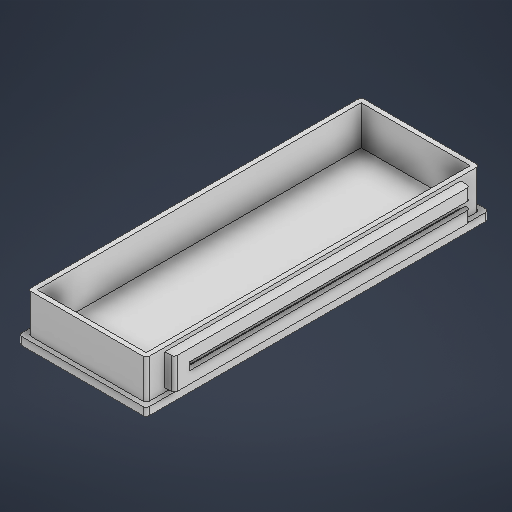
# Autodesk Inventor part: module_command
Saved by Autodesk Inventor 2025.2 (Build 292293000, 293)
## iProperties
Created: 2025-09-05
Part Number: module_command
Material: Generic
Document SubType Name: Modeling
Designer: sam
Density: 1 g/cm^3
Appearance: Default
Author: sam
Autodesk Inventor part; units mm, degrees
ref_plane "YZ Plane" through (0, 0, 0) normal (1, 0, 0) x (0, 1, 0)
ref_plane "XZ Plane" through (0, 0, 0) normal (0, 1, 0) x (-1, 0, 0)
ref_plane "XY Plane" through (0, 0, 0) normal (0, 0, 1) x (1, 0, 0)
sketch "Sketch1" plane through (0, 0, 0) normal (0, 1, 0) x (-1, 0, 0)
  line L0 (-41, -110) -> (41, -110)
  line L1 (41, -110) -> (41, 110)
  line L2 (41, 110) -> (-41, 110)
  line L3 (-41, 110) -> (-41, -110)
  line L4 (-41, -110) -> (41, 110) construction
  line L5 (41, -110) -> (-41, 110) construction
  point P0 (0, 0)
  dimension "d0" = 82
  dimension "d1" = 220
  constraints: 12 end point, 2 midpoint, 2 parallel, 1 horizontal, 1 perpendicular
  measures "d0" distance of L2.end L1.end
  measures "d1" distance of L1.end L0.end
extrude "Extrusion1" add sketch "Sketch1" along normal blind 5
sketch "Sketch2" plane through (0, 5, 0) normal (0, 1, 0) x (1, 0, 0)
  line L0 (-41, 110) -> (-41, -110) projected
  line L1 (-41, -110) -> (41, -110) projected
  line L2 (41, -110) -> (41, 110) projected
  line L3 (41, 110) -> (-41, 110) projected
  line L4 (38, 107) -> (-38, 107)
  line L5 (-38, 107) -> (-38, -107)
  line L6 (-38, -107) -> (38, -107)
  line L7 (38, -107) -> (38, 107)
  line L8 (38, 107) -> (-38, -107) construction
  line L9 (-38, 107) -> (38, -107) construction
  line L10 (35, 104) -> (-35, 104)
  line L11 (-35, 104) -> (-35, -104)
  line L12 (-35, -104) -> (35, -104)
  line L13 (35, -104) -> (35, 104)
  line L14 (35, 104) -> (-35, -104) construction
  line L15 (-35, 104) -> (35, -104) construction
  point P0 (0, 0)
  dimension "d4" = 3
  dimension "d5" = 3
  dimension "d6" = 3
  dimension "d7" = 3
  constraints: 24 end point, 4 midpoint, 4 parallel, 2 horizontal, 2 perpendicular
  measures "d4" distance between parallel lines of L0 L5
  measures "d5" distance between parallel lines of L1 L6
  measures "d6" distance between parallel lines of L5 L11
  measures "d7" distance between parallel lines of L6 L12
extrude "Extrusion2" add sketch "Sketch2" along normal blind 25 contours L7 L6 L5 L4
fillet "Fillet1" radius 2 4 edges at (-38, 17.5, 107) (38, 17.5, 107) (38, 17.5, -107) (-38, 17.5, -107)
fillet "Fillet2" radius 2 4 edges at (-41, 2.5, 110) (41, 2.5, 110) (41, 2.5, -110) (-41, 2.5, -110)
sketch "Sketch3" plane through (38, 5, 105) normal (1, 0, 0) x (0, 0, -1)
  line L0 (210, 25) -> (210, 0) projected
  line L1 (0, 25) -> (210, 25) projected
  line L2 (0, 0) -> (0, 25) projected
  line L3 (210, 0) -> (0, 0) projected
  line L4 (10, 22.5) -> (200, 22.5)
  line L5 (200, 22.5) -> (200, 2.5)
  line L6 (200, 2.5) -> (10, 2.5)
  line L7 (10, 2.5) -> (10, 22.5)
  point P0 (105, -5)
  dimension "d12" = 10
  dimension "d14" = 10
  dimension "d15" = 2.5
  dimension "d16" = 2.5
  constraints: 8 end point, 2 parallel, 1 horizontal, 1 perpendicular
  measures "d12" distance between parallel lines of L2 L7
  measures "d14" distance between parallel lines of L0 L5
  measures "d15" distance between parallel lines of L1 L4
  measures "d16" distance between parallel lines of L3 L6
extrude "Extrusion3" add sketch "Sketch3" along normal blind 6 contours L4 L5 L6 L7
sketch "Sketch4" plane through (38, 7.5, -95) normal (0, 0, -1) x (-1, 0, 0)
  line L0 (0, 20) -> (0, 0) projected
  line L1 (0, 20) -> (-6, 20) projected
  line L2 (-6, 0) -> (-6, 20) projected
  line L3 (0, 0) -> (-6, 0) projected
  line L4 (-6, 0) -> (-6, 20) projected
  line L5 (-6, 12.5) -> (-3, 12.5)
  line L6 (-3, 12.5) -> (-3, 7.5)
  line L7 (-3, 7.5) -> (-6, 7.5)
  line L8 (-6, 7.5) -> (-6, 12.5)
  line L9 (0, -2.5) -> (0, 22.5) projected
  line L10 (0, 15) -> (-3, 15)
  line L11 (-3, 15) -> (-3, 5)
  line L12 (-3, 5) -> (0, 5)
  line L13 (0, 5) -> (0, 15)
  point P0 (38, -7.5)
  point P1 (-4.5, 12.5)
  point P2 (-6, 7.5)
  point P3 (-3, 7.5)
  point P4 (0, 5)
  point P5 (-3, 12.5)
  dimension "d19" = 3
  dimension "d20" = 7.5
  dimension "d21" = 7.5
  dimension "d22" = 5
  dimension "d23" = 5
  constraints: 16 end point, 4 parallel, 3 point on line, 2 horizontal, 2 perpendicular, 1 midpoint
  measures "d19" distance of L6.end L7.end
  measures "d20" distance from line of L1 point (-4.5, 12.5)
  measures "d21" distance between parallel lines of L3 L7
  measures "d22" distance between parallel lines of L3 L12
  measures "d23" distance between parallel lines of L1 L10
extrude "Extrusion4" cut sketch "Sketch4" against normal blind 180 contours L0 L12 L11 L6 L10 | L5 L6 L7 L2
fillet "Fillet3" radius 2 3 edges at (44, 17.5, 95) (44, 11.25, -95) (44, 23.75, -95)
body "Solid1"
